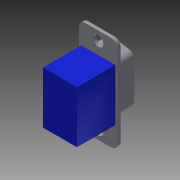
# Autodesk Inventor part: anschluss_daten_2
Saved by Autodesk Inventor 2015 (Build 190159000, 159)
## iProperties
Created: 2018-04-03
Part Number: anschluss_daten_2
Material: Generisch
Document SubType Name: Modeling
Designer: wepet
Density: 1 g/cm^3
Appearance: Vorgabe
Author: wepet
Autodesk Inventor part; units mm, degrees
ref_plane "YZ Plane" through (0, 0, 0) normal (1, 0, 0) x (0, 1, 0)
ref_plane "XZ Plane" through (0, 0, 0) normal (0, 1, 0) x (-1, 0, 0)
ref_plane "XY Plane" through (0, 0, 0) normal (0, 0, 1) x (1, 0, 0)
sketch "Skizze9" plane through (0, 0, 0) normal (0, 1, 0) x (-1, 0, 0)
  line L0 (4.275, 15.405) -> (-4.275, 15.405)
  line L1 (-6.275, 13.405) -> (-6.275, -13.405)
  line L2 (-4.275, -15.405) -> (4.275, -15.405)
  line L3 (6.275, -13.405) -> (6.275, 13.405)
  line L4 (0, 0) -> (0, -15.405) construction
  line L5 (0, 0) -> (6.275, 0) construction
  arc A0 (6.275, 13.405) -> (4.275, 15.405) centre (4.275, 13.405) ccw
  arc A1 (-6.275, -13.405) -> (-4.275, -15.405) centre (-4.275, -13.405) ccw
  arc A2 (4.275, -15.405) -> (6.275, -13.405) centre (4.275, -13.405) ccw
  arc A3 (-4.275, 15.405) -> (-6.275, 13.405) centre (-4.275, 13.405) ccw
  point P0 (6.275, 15.405)
  point P1 (-6.275, -15.405)
  point P2 (-6.275, 15.405)
  point P3 (6.275, -15.405)
  dimension "d41" = 30.81
  dimension "d42" = 12.55
  dimension "d61" = 2
  constraints: 12 end point, 8 point on circle, 8 point on line, 8 tangent, 4 centre point, 3 equal radius, 3 perpendicular, 2 midpoint, 2 parallel, 1 horizontal
  measures "d41" distance of point (6.275, -15.405) point (6.275, 15.405)
  measures "d42" distance of point (6.275, 15.405) point (-6.275, 15.405)
  measures "d61" radius of A0
extrude "Extrusion6" add sketch "Skizze9" along normal blind 1
sketch "Skizze10" plane through (0, 1, 0) normal (0, 1, 0) x (1, 0, 0)
  line L0 (-4.275, -15.405) -> (4.275, -15.405) projected
  line L1 (6.275, -13.405) -> (6.275, 13.405) projected
  line L2 (4.275, 15.405) -> (-4.275, 15.405) projected
  line L3 (-6.275, 13.405) -> (-6.275, -13.405) projected
  line L4 (4.6, -6.0831) -> (4.6, 6.0831)
  line L5 (2.9473, 8.0527) -> (-2.2527, 8.9696)
  line L6 (-4.6, 7) -> (-4.6, -7)
  line L7 (-2.2527, -8.9696) -> (2.9473, -8.0527)
  line L8 (0, 0) -> (-4.6, 0) construction
  line L9 (0, 0) -> (4.6, 0) construction
  line L10 (-4.6, -9.3835) -> (6.275, -9.3835) construction
  line L11 (-4.6, 9.3835) -> (6.275, 9.3835) construction
  arc A0 (-4.6, -7) -> (-2.2527, -8.9696) centre (-2.6, -7) ccw
  arc A1 (-2.2527, 8.9696) -> (-4.6, 7) centre (-2.6, 7) ccw
  arc A2 (2.9473, -8.0527) -> (4.6, -6.0831) centre (2.6, -6.0831) ccw
  arc A3 (4.6, 6.0831) -> (2.9473, 8.0527) centre (2.6, 6.0831) ccw
  arc A4 (4.275, -15.405) -> (6.275, -13.405) centre (4.275, -13.405) ccw projected
  arc A5 (6.275, 13.405) -> (4.275, 15.405) centre (4.275, 13.405) ccw projected
  arc A6 (-4.275, 15.405) -> (-6.275, 13.405) centre (-4.275, 13.405) ccw projected
  arc A7 (-6.275, -13.405) -> (-4.275, -15.405) centre (-4.275, -13.405) ccw projected
  dimension "d45" = 10
  dimension "d46" = 4.6
  dimension "d47" = 4.6
  dimension "d49" = 2
  dimension "d67" = 14
  dimension "d68" = 18
  constraints: 16 end point, 8 point on circle, 8 tangent, 6 point on line, 4 centre point, 4 perpendicular, 3 equal radius, 2 midpoint, 1 parallel, 1 vertical
  measures "d45" angle of L10 L7
  measures "d46" distance of L8.start L8.end
  measures "d47" distance of L8.start L9.end
  measures "d49" radius of A0
  measures "d67" distance of A1.centre A0.centre
extrude "Extrusion7" add sketch "Skizze10" along normal blind 6.1 contours A2 L7 A0 L6 A1 L5 A3 L4
sketch "Skizze11" plane through (0, 1, 0) normal (0, 1, 0) x (1, 0, 0)
  arc A0 (-2.2527, 8.9696) -> (-4.6, 7) centre (-2.6, 7) ccw projected
  line L0 (-2.2527, 8.9696) -> (2.9473, 8.0527) projected
  arc A1 (4.6, 6.0831) -> (2.9473, 8.0527) centre (2.6, 6.0831) ccw projected
  line L1 (4.6, 6.0831) -> (4.6, -6.0831) projected
  arc A2 (2.9473, -8.0527) -> (4.6, -6.0831) centre (2.6, -6.0831) ccw projected
  line L2 (2.9473, -8.0527) -> (-2.2527, -8.9696) projected
  arc A3 (-4.6, -7) -> (-2.2527, -8.9696) centre (-2.6, -7) ccw projected
  line L3 (-4.6, -7) -> (-4.6, 7) projected
  line L4 (-4.275, -15.405) -> (4.275, -15.405) projected
  line L5 (6.275, -13.405) -> (6.275, 13.405) projected
  line L6 (4.275, 15.405) -> (-4.275, 15.405) projected
  line L7 (-6.275, 13.405) -> (-6.275, -13.405) projected
  line L8 (0, 0) -> (0, 12.5) construction
  line L9 (0, 0) -> (0, -12.5) construction
  arc A4 (4.275, -15.405) -> (6.275, -13.405) centre (4.275, -13.405) ccw projected
  arc A5 (6.275, 13.405) -> (4.275, 15.405) centre (4.275, 13.405) ccw projected
  arc A6 (-4.275, 15.405) -> (-6.275, 13.405) centre (-4.275, 13.405) ccw projected
  arc A7 (-6.275, -13.405) -> (-4.275, -15.405) centre (-4.275, -13.405) ccw projected
  dimension "d52" = 12.5
  dimension "d53" = 12.5
  constraints: 4 end point, 2 coincident, 2 vertical
  measures "d52" distance of L8.start L8.end
  measures "d53" distance of L8.start L9.end
hole "Bohrung3" at (0, 1, 12.5) at (0, 1, -12.5) direction (0, -1, 0) diameter 3.3 end through all
sketch "Skizze12" plane through (0, 0, 0) normal (0, -1, 0) x (1, 0, 0)
  circle A0 centre (0, 12.5) radius 1.65 projected
  circle A1 centre (0, -12.5) radius 1.65 projected
  line L0 (-4.275, 15.405) -> (4.275, 15.405) projected
  arc A2 (-4.275, 15.405) -> (-6.275, 13.405) centre (-4.275, 13.405) ccw projected
  line L1 (-6.275, -13.405) -> (-6.275, 13.405) projected
  arc A3 (-6.275, -13.405) -> (-4.275, -15.405) centre (-4.275, -13.405) ccw projected
  line L2 (4.275, -15.405) -> (-4.275, -15.405) projected
  arc A4 (4.275, -15.405) -> (6.275, -13.405) centre (4.275, -13.405) ccw projected
  line L3 (6.275, 13.405) -> (6.275, -13.405) projected
  arc A5 (6.275, 13.405) -> (4.275, 15.405) centre (4.275, 13.405) ccw projected
  line L4 (-5.55, -8.46) -> (5.55, -8.46)
  line L5 (5.55, -8.46) -> (5.55, 8.46)
  line L6 (5.55, 8.46) -> (-5.55, 8.46)
  line L7 (-5.55, 8.46) -> (-5.55, -8.46)
  line L8 (0, 0) -> (0, 8.46) construction
  line L9 (0, 0) -> (-5.55, 0) construction
  dimension "d62" = 11.1
  dimension "d63" = 16.92
  constraints: 12 end point, 3 perpendicular, 2 midpoint, 2 parallel, 1 horizontal
  measures "d62" distance of L4.start L4.end
  measures "d63" distance of L6.end L4.start
extrude "Extrusion8" add sketch "Skizze12" along normal blind 12.5 contours L7 L6 L5 L4
